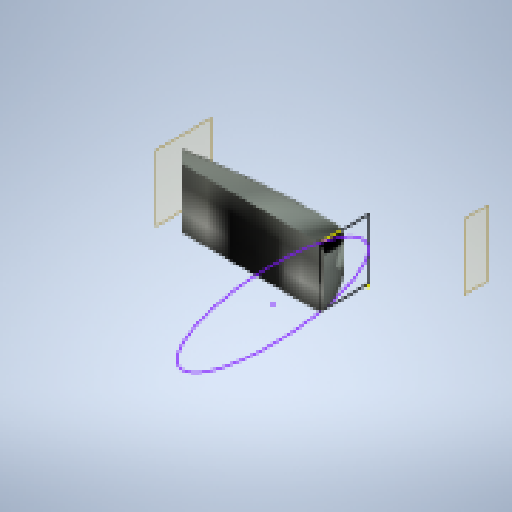
# Autodesk Inventor part: Part2
Saved by Autodesk Inventor 2025.2 (Build 292293000, 293)
## iProperties
Created: 2024-12-25
Part Number: Part2
Material: Generic
Document SubType Name: Modeling
Designer: naka6
Density: 1 g/cm^3
Appearance: 型枠 穴
Author: naka6
Autodesk Inventor part; units mm, degrees
ref_plane "YZ Plane" through (0, 0, 0) normal (1, 0, 0) x (0, 1, 0)
ref_plane "XZ Plane" through (0, 0, 0) normal (0, 1, 0) x (-1, 0, 0)
ref_plane "XY Plane" through (0, 0, 0) normal (0, 0, 1) x (1, 0, 0)
sketch "スケッチ1" plane through (0, 0, 0) normal (0, 0, 1) x (1, 0, 0)
  line L0 (0, 0) -> (-67, 0)
  line L1 (-67, 0) -> (-67, 25.348127)
  line L2 (-67, 25.348127) -> (0, 25.348127)
  line L3 (0, 25.348127) -> (0, 0)
  line L4 (-2, 25.348127) -> (-58, 25.348127)
  line L5 (-67, 19.989971) -> (-67, 6.24001)
  arc A0 (-64.160911, 23.817801) -> (-67, 19.989971) centre (-63, 19.989971) ccw
  ellipse E0 centre (-39, 13.11499) end of major axis (0, 13.11499) minor radius 14.007913 (-58, 25.348127) -> (-64.160911, 23.817801) ccw
  arc A1 (-67, 6.24001) -> (-65.173197, 2.881853) centre (-63, 6.24001) ccw
  ellipse E1 centre (-39, 13.11499) end of major axis (0, 13.11499) minor radius 14.007913 (-64.160911, 2.412179) -> (-58, 0.881853) ccw
  line L6 (-58, 0.881853) -> (-2, 0.881853)
  spline S0 degree 3 poles (-2, 0.881853) (-1.744334, 0.881853) (-1.491388, 0.931844) (-1.015757, 1.126636) (-0.798365, 1.270338) (-0.42569, 1.635842) (-0.275413, 1.855583) (-0.114451, 2.227344) (-0.071754, 2.362557) (-0.017195, 2.626393) (-0.002908, 2.753901) (-0.0004, 2.881853) knots 0 0 0 0 0.24426495 0.24426495 0.49099805 0.49099805 0.74278466 0.74278466 0.87777234 0.87777234 1 1 1 1
  spline S1 degree 3 poles (0, 23.30727) (0, 23.578351) (-0.05287, 23.847124) (-0.257931, 24.345436) (-0.407121, 24.570982) (-0.780649, 24.946663) (-0.999731, 25.094657) (-1.481819, 25.296217) (-1.739471, 25.348127) (-2, 25.348127) knots 0 0 0 0 0.2552907 0.2552907 0.5075389 0.5075389 0.75443111 0.75443111 1 1 1 1
  line L7 (0, 2.92271) -> (0, 23.30727)
  arc A2 (-65.173197, 2.881853) -> (-64.160911, 2.412179) centre (-63, 6.24001) ccw
  line L8 (-67, 0.881853) -> (0, 0.881853)
  spline S2 degree 3 poles (-2, 0.881853) (-1.744334, 0.881853) (-1.491388, 0.931844) (-1.015757, 1.126636) (-0.798365, 1.270338) (-0.42569, 1.635842) (-0.275413, 1.855583) (-0.114451, 2.227344) (-0.071754, 2.362557) (-0.017195, 2.626393) (-0.002908, 2.753901) (-0.0004, 2.881853) knots 0 0 0 0 0.24426495 0.24426495 0.49099805 0.49099805 0.74278466 0.74278466 0.87777234 0.87777234 1 1 1 1
  line L9 (0, 2.92271) -> (0, 23.30727)
  line L10 (-58, 0.881853) -> (-2, 0.881853)
  circle A3 centre (-2, 2.92271) radius 2.025797
  point P0 (-0.776, 1.308498)
  point P1 (0, 2.600445)
  constraints: 10 end point, 5 point on line, 2 parallel, 1 centre point, 1 horizontal, 1 perpendicular, 3 other
extrude "押し出し1" add sketch "スケッチ1" along normal blind 20 contours A3 S0 L3 | L6 E1 A2 A1 L1 A0 E0 L2 S1 L3 A3 S0 | S0 A3 L3
sketch "スケッチ2" plane through (-58, 0.881853, 0) normal (0, -1, 0) x (1, 0, 0)
  line L0 (-9, 0) -> (-9, 20)
  line L1 (0, 0) -> (56, 0)
  line L2 (0, 20) -> (56, 20)
  circle A0 centre (38, 20) radius 20
  line L3 (58, 0) -> (58, 20)
  line L4 (-23, 11) -> (-9, 11)
  line L5 (-9, 11) -> (35.568366, 0)
  line L6 (0, 20) -> (-6.160911, 13.839089)
  line L7 (-7.173197, 12.826803) -> (-9, 11)
  line L8 (-6.160911, 13.839089) -> (-7.173197, 12.826803)
  line L9 (0, 0) -> (-6.160911, 0)
  line L10 (-6.160911, 0) -> (-9, 0)
  line L11 (0, 20) -> (-6.160911, 20)
  line L12 (-6.160911, 20) -> (-9, 20)
  line L13 (57.224, 0) -> (56, 0)
  line L14 (58, 0) -> (57.224, 0)
  point P0 (38, 0)
  constraints: 3 tangent, 2 end point, 2 point on line, 1 centre point
extrude "押し出し2" cut sketch "スケッチ2" against normal through all contours L0 L5 L1 L9 L10 | L0 L12 L11 L6 L8 L7 | A0 L3 L14 L13 L1
ref_plane "作業平面3" through (-1.999992, 0.881853, 11.282218) normal (1, 0.0000003, 0) x (-0.0000003, 1, -0.0000007)
sketch "スケッチ5" plane through (-1.999992, 0.881853, 11.282218) normal (1, 0.0000003, 0) x (-0.0000003, 1, -0.0000007)
  line L0 (0.000014, -11.282218) -> (0.000014, -11.282218)
  line L1 (24.466274, 0) -> (24.466268, 8.717798)
  line L2 (0.000014, -11.282218) -> (24.466268, -11.282218)
  line L3 (24.466268, -11.282218) -> (24.466268, 8.717798)
  line L4 (24.466268, 8.717798) -> (0.000014, 8.717798)
  line L5 (0.000014, 8.717798) -> (0.000014, -11.282218)
  ellipse E0 centre (12.233141, 27.591175) end of major axis (12.233141, -11.282218) minor radius 13.993003
  point P0 (-0.881847, -11.282219)
  point P1 (12.233141, -11.282218)
  point P2 (24.466274, 0)
  constraints: 8 end point, 2 horizontal, 2 parallel, 1 perpendicular, 4 other
extrude "押し出し3" cut sketch "スケッチ5" against normal blind 100 contours L3 L2 E0 L1 | E0 L2 L5
sketch "スケッチ6" plane through (-1.999992, 0.881853, 11.282218) normal (-1, -0.0000003, 0) x (0, 0.0000007, 1)
  line L0 (0, 0) -> (0, 2.376004)
  line L1 (-0.000016, 0) -> (8.717782, -0.000006)
  ellipse E0 centre (27.591175, 12.233141) end of major axis (66.464569, 12.233141) minor radius 13.993003 (0, 2.376004) -> (8.717782, -0.000006) ccw
  line L2 (0, 22.090278) -> (0, 24.466274)
  ellipse E1 centre (27.591175, 12.233141) end of major axis (66.464569, 12.233141) minor radius 13.993003 (8.717798, 24.466268) -> (0, 22.090278) ccw
  line L3 (0, 24.466274) -> (8.717798, 24.466268)
  point P0 (-11.282219, -0.881847)
  constraints: 2 other
extrude "押し出し4" cut sketch "スケッチ6" against normal blind 100 contours L2 L3 E1
extrude "押し出し5" cut sketch "スケッチ5" along normal blind 100 contours E0 L2 L5
fillet "フィレット1" radius 4 2 edges at (-43.7049, 6.0921, 5.2505) (-43.7049, 20.1379, 5.2505)
fillet "フィレット2" radius 3 4 edges at (-1.0413, 23.7564, 13.6306) (-10.0911, 8.0581, 2.6272) (-10.0911, 18.1719, 2.6272) (-1.0353, 2.468, 13.6487)
ref_plane "作業平面4" through (-67, 10.435912, 11) normal (1, 0, 0) x (0, 1, 0)
